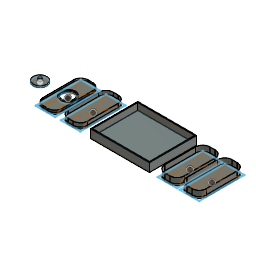
insert_test (Autodesk Fusion 360 design; units mm, degrees)
Autodesk Fusion 360 part; units mm, degrees
sketch "Sketch1" plane through (0, 0, 0) normal (0, 1, 0) x (1, 0, 0)
  line L0 (163.5, 131) -> (-163.5, 131)
  line L1 (-163.5, 131) -> (-163.5, -131)
  line L2 (-163.5, -131) -> (163.5, -131)
  line L3 (163.5, -131) -> (163.5, 131)
  line L4 (163.5, 131) -> (-163.5, -131) construction
  line L5 (-163.5, 131) -> (163.5, -131) construction
  line L6 (158.5, 126) -> (-158.5, 126)
  line L7 (-158.5, 126) -> (-158.5, -126)
  line L8 (-158.5, -126) -> (158.5, -126)
  line L9 (158.5, -126) -> (158.5, 126)
  line L10 (158.5, 126) -> (-158.5, -126) construction
  line L11 (-158.5, 126) -> (158.5, -126) construction
  dimension "d1" = 327
  dimension "d2" = 262
  dimension "d3" = 317
  dimension "d4" = 252
  constraint horizontal L0
  constraint perpendicular L0 L1
  constraint parallel L0 L2
  constraint parallel L1 L3
  constraint coincident L4 origin
  constraint coincident L5 origin
  constraint horizontal L6
  constraint perpendicular L6 L7
  constraint parallel L6 L8
  constraint parallel L7 L9
  constraint coincident L10 origin
  constraint coincident L11 origin
  measures "d1" distance of L1.end L2.end
  measures "d2" distance of L0.end L1.end
  measures "d3" distance of L7.end L8.end
  measures "d4" distance of L6.end L7.end
extrude "Extrude1" add sketch "Sketch1" along normal blind 48 makes body 1
sketch "Sketch2" plane through (0, 0, 0) normal (0, 1, 0) x (1, 0, 0)
  line L0 (-161.5, 130) -> (161.5, 130)
  line L1 (161.5, 130) -> (161.5, -130)
  line L2 (161.5, -130) -> (-161.5, -130)
  line L3 (-161.5, -130) -> (-161.5, 130)
  line L4 (-161.5, 130) -> (161.5, -130) construction
  line L5 (161.5, 130) -> (-161.5, -130) construction
  dimension "d7" = 323
  dimension "d8" = 260
  constraint horizontal L0
  constraint perpendicular L0 L1
  constraint parallel L0 L2
  constraint parallel L1 L3
  constraint coincident L4 origin
  constraint coincident L5 origin
  measures "d7" distance of L1.end L2.end
  measures "d8" distance of L0.end L1.end
extrude "Extrude2" add sketch "Sketch2" along normal blind 10 bodies 1
sketch "Sketch3" plane through (0, 10, 0) normal (0, 1, 0) x (-1, 0, 0)
  line L0 (158.5, 126) -> (-158.5, 126)
  line L1 (-158.5, 126) -> (-158.5, -126)
  line L2 (-158.5, -126) -> (158.5, -126)
  line L3 (158.5, -126) -> (158.5, 126)
sketch "Sketch4" plane through (0, 10, 0) normal (0, 1, 0) x (-1, 0, 0)
  line L0 (158.5, 126) -> (-158.5, 126)
  line L1 (-158.5, 126) -> (-158.5, -126)
  line L2 (-158.5, -126) -> (158.5, -126)
  line L3 (158.5, -126) -> (158.5, 126)
  line L4 (-320, -124) -> (-220, -124)
  line L5 (-220, -124) -> (-220, 124)
  line L6 (-220, 124) -> (-320, 124)
  line L7 (-320, 124) -> (-320, -124)
  line L8 (-320, -124) -> (-220, 124) construction
  line L9 (-220, -124) -> (-320, 124) construction
  point P0 (-270, 0)
  dimension "d17" = 100
  dimension "d18" = 248
  constraint horizontal L4
  constraint perpendicular L4 L5
  constraint parallel L4 L6
  constraint parallel L5 L7
  constraint coincident L8 P0
  constraint coincident L9 P0
  measures "d17" distance of L5.end L6.end
  measures "d18" distance of L4.end L5.end
sketch "Sketch5" plane through (0, 20, 0) normal (0, 1, 0) x (-1, 0, 0)
sketch "Sketch6" plane through (0, 10, 0) normal (0, 1, 0) x (-1, 0, 0)
  line L0 (158.5, 126) -> (-158.5, 126)
  line L1 (-158.5, 126) -> (-158.5, -126)
  line L2 (-158.5, -126) -> (158.5, -126)
  line L3 (158.5, -126) -> (158.5, 126)
sketch "Sketch9" plane through (0, 20, 0) normal (0, 1, 0) x (-1, 0, 0)
sketch "Sketch10" plane through (0, 10, 0) normal (0, 1, 0) x (-1, 0, 0)
sketch "Sketch11" plane through (0, 0, 0) normal (0, 1, 0) x (1, 0, 0)
sketch "Sketch12" plane through (0, 20, 0) normal (0, 1, 0) x (1, 0, 0)
sketch "Sketch14" plane through (0, 0, 0) normal (0, 1, 0) x (1, 0, 0)
sketch "Sketch15" plane through (0, 0, 0) normal (0, 1, 0) x (1, 0, 0)
  line L0 (207.402, 121.291) -> (316.402, 121.291)
  line L1 (316.402, 121.291) -> (316.402, -130.109)
  line L2 (316.402, -130.109) -> (207.402, -130.109)
  line L3 (207.402, -130.109) -> (207.402, 121.291)
  line L4 (207.402, 121.291) -> (316.402, -130.109) construction
  line L5 (316.402, 121.291) -> (207.402, -130.109) construction
  line L6 (315.802, 120.691) -> (208.002, 120.691)
  line L7 (208.002, 120.691) -> (208.002, -129.509)
  line L8 (208.002, -129.509) -> (315.802, -129.509)
  line L9 (315.802, -129.509) -> (315.802, 120.691)
  line L10 (315.802, 120.691) -> (208.002, -129.509) construction
  line L11 (208.002, 120.691) -> (315.802, -129.509) construction
  point P0 (261.902, -4.409)
  point P1 (261.902, -4.409)
  dimension "d42" = 109
  dimension "d43" = 251.4
  dimension "d44" = 107.8
  dimension "d45" = 250.2
  constraint horizontal L0
  constraint perpendicular L0 L1
  constraint parallel L0 L2
  constraint parallel L1 L3
  constraint coincident L4 P1
  constraint coincident L5 P1
  constraint horizontal L6
  constraint perpendicular L6 L7
  constraint parallel L6 L8
  constraint parallel L7 L9
  constraint coincident L10 P1
  constraint coincident L11 P1
  constraint coincident P1 P0
  measures "d42" distance of L1.end L2.end
  measures "d43" distance of L0.end L1.end
  measures "d44" distance of L7.end L8.end
  measures "d45" distance of L6.end L7.end
extrude "Extrude8" add sketch "Sketch15" along normal blind 40 separate body makes body 2
extrude "Extrude9" add sketch "Sketch15" along normal blind 10 contours L6 L7 L8 L9 bodies 2
sketch "Sketch16" plane through (0, 0, 0) normal (0, 1, 0) x (1, 0, 0)
sketch "Sketch17" plane through (0, 0, 0) normal (0, 1, 0) x (1, 0, 0)
  line L0 (329.9494, 121.3227) -> (438.9494, 121.3227)
  line L1 (438.9494, 121.3227) -> (438.9494, -130.0773)
  line L2 (438.9494, -130.0773) -> (329.9494, -130.0773)
  line L3 (329.9494, -130.0773) -> (329.9494, 121.3227)
  line L4 (329.9494, 121.3227) -> (438.9494, -130.0773) construction
  line L5 (438.9494, 121.3227) -> (329.9494, -130.0773) construction
  line L6 (438.3494, 120.7227) -> (330.5494, 120.7227)
  line L7 (330.5494, 120.7227) -> (330.5494, -129.4773)
  line L8 (330.5494, -129.4773) -> (438.3494, -129.4773)
  line L9 (438.3494, -129.4773) -> (438.3494, 120.7227)
  line L10 (438.3494, 120.7227) -> (330.5494, -129.4773) construction
  line L11 (330.5494, 120.7227) -> (438.3494, -129.4773) construction
  point P0 (384.4494, -4.3773)
  point P1 (384.4494, -4.3773)
  dimension "d50" = 109
  dimension "d51" = 251.4
  dimension "d52" = 107.8
  dimension "d53" = 250.2
  constraint horizontal L0
  constraint perpendicular L0 L1
  constraint parallel L0 L2
  constraint parallel L1 L3
  constraint coincident L4 P1
  constraint coincident L5 P1
  constraint horizontal L6
  constraint perpendicular L6 L7
  constraint parallel L6 L8
  constraint parallel L7 L9
  constraint coincident L10 P1
  constraint coincident L11 P1
  constraint coincident P1 P0
  measures "d50" distance of L1.end L2.end
  measures "d51" distance of L0.end L1.end
  measures "d52" distance of L7.end L8.end
  measures "d53" distance of L6.end L7.end
sketch "Sketch18" plane through (0, 0, 0) normal (0, 1, 0) x (1, 0, 0)
  line L0 (434.5, 120.7) -> (325.5, 120.7)
  line L1 (325.5, 120.7) -> (325.5, -120.7)
  line L2 (325.5, -120.7) -> (434.5, -120.7)
  line L3 (434.5, -120.7) -> (434.5, 120.7)
  line L4 (434.5, 120.7) -> (325.5, -120.7) construction
  line L5 (325.5, 120.7) -> (434.5, -120.7) construction
  point P0 (380, 0)
  dimension "d54" = 109
  dimension "d55" = 241.4
  constraint horizontal L0
  constraint perpendicular L0 L1
  constraint parallel L0 L2
  constraint parallel L1 L3
  constraint coincident L4 P0
  constraint coincident L5 P0
  measures "d54" distance of L1.end L2.end
  measures "d55" distance of L0.end L1.end
sketch "Sketch20" plane through (0, 0, 0) normal (0, 1, 0) x (1, 0, 0)
  line L0 (-225.9, 125.7) -> (-334.5, 125.7)
  line L1 (-334.5, 125.7) -> (-334.5, -125.5)
  line L2 (-334.5, -125.5) -> (-225.9, -125.5)
  line L3 (-225.9, -125.5) -> (-225.9, 125.7)
  line L4 (-225.9, 125.7) -> (-334.5, -125.5) construction
  line L5 (-334.5, 125.7) -> (-225.9, -125.5) construction
  point P0 (-280.2, 0.1)
  dimension "d60" = 108.6
  dimension "d61" = 251.2
  constraint horizontal L0
  constraint perpendicular L0 L1
  constraint parallel L0 L2
  constraint parallel L1 L3
  constraint coincident L4 P0
  constraint coincident L5 P0
  measures "d60" distance of L1.end L2.end
  measures "d61" distance of L0.end L1.end
sketch "Sketch35" plane through (0, 0, 0) normal (0, 1, 0) x (1, 0, 0)
  line L0 (-365.7, 125.7) -> (-474.3, 125.7)
  line L1 (-474.3, 125.7) -> (-474.3, -125.7)
  line L2 (-474.3, -125.7) -> (-365.7, -125.7)
  line L3 (-365.7, -125.7) -> (-365.7, 125.7)
  line L4 (-365.7, 125.7) -> (-474.3, -125.7) construction
  line L5 (-474.3, 125.7) -> (-365.7, -125.7) construction
  circle A0 centre (-420, 0) radius 37.5
  point P0 (-420, 0)
  dimension "d73" = 108.6
  dimension "d82" = 75
  dimension "d111" = 251.4
  constraint horizontal L0
  constraint perpendicular L0 L1
  constraint parallel L0 L2
  constraint parallel L1 L3
  constraint coincident L4 P0
  constraint coincident L5 P0
  constraint coincident P0 A0.centre
  measures "d73" distance of L1.end L2.end
  measures "d82" diameter of A0
  measures "d111" distance of L0.end L1.end
sketch "Sketch37" plane through (0, 0, 0) normal (0, 1, 0) x (1, 0, 0)
  line L0 (-366.8902, 125.3136) -> (-473.6902, 125.3136)
  line L1 (-473.6902, 125.3136) -> (-473.6902, -124.8864)
  line L2 (-473.6902, -124.8864) -> (-366.8902, -124.8864)
  line L3 (-366.8902, -124.8864) -> (-366.8902, 125.3136)
  line L4 (-366.8902, 125.3136) -> (-473.6902, -124.8864) construction
  line L5 (-473.6902, 125.3136) -> (-366.8902, -124.8864) construction
  line L6 (-367.5902, 124.6136) -> (-472.9902, 124.6136)
  line L7 (-472.9902, 124.6136) -> (-472.9902, -124.1864)
  line L8 (-472.9902, -124.1864) -> (-367.5902, -124.1864)
  line L9 (-367.5902, -124.1864) -> (-367.5902, 124.6136)
  line L10 (-367.5902, 124.6136) -> (-472.9902, -124.1864) construction
  line L11 (-472.9902, 124.6136) -> (-367.5902, -124.1864) construction
  point P0 (-420.2902, 0.2136)
  point P1 (-420.2902, 0.2136)
  dimension "d76" = 106.8
  dimension "d77" = 250.2
  dimension "d78" = 105.4
  dimension "d79" = 248.8
  constraint horizontal L0
  constraint perpendicular L0 L1
  constraint parallel L0 L2
  constraint parallel L1 L3
  constraint coincident L4 P1
  constraint coincident L5 P1
  constraint horizontal L6
  constraint perpendicular L6 L7
  constraint parallel L6 L8
  constraint parallel L7 L9
  constraint coincident L10 P1
  constraint coincident L11 P1
  constraint coincident P1 P0
  measures "d76" distance of L1.end L2.end
  measures "d77" distance of L0.end L1.end
  measures "d78" distance of L7.end L8.end
  measures "d79" distance of L6.end L7.end
extrude "Extrude14" add sketch "Sketch37" along normal blind 20 separate body makes body 3
sketch "Sketch38" plane through (0, 0, 0) normal (0, 1, 0) x (1, 0, 0)
extrude "Extrude15" add sketch "Sketch35" along normal blind 10 bodies 3
sketch "Sketch39" plane through (0, 0, 0) normal (0, 1, 0) x (1, 0, 0)
sketch "Sketch40" plane through (0, 0, 0) normal (0, 0, 1) x (1, 0, 0)
sketch "Sketch41" plane through (0, 0, 0) normal (0, 1, 0) x (1, 0, 0)
sketch "Sketch42" plane through (0, 0, 0) normal (0, 1, 0) x (1, 0, 0)
  line L0 (-226.5, 125.1) -> (-333.9, 125.1)
  line L1 (-333.9, 125.1) -> (-333.9, -125.1)
  line L2 (-333.9, -125.1) -> (-226.5, -125.1)
  line L3 (-226.5, -125.1) -> (-226.5, 125.1)
  line L4 (-226.5, 125.1) -> (-333.9, -125.1) construction
  line L5 (-333.9, 125.1) -> (-226.5, -125.1) construction
  line L6 (-225.8538, 125.6801) -> (-334.5462, 125.6801)
  line L7 (-334.5462, 125.6801) -> (-334.5462, -125.6801)
  line L8 (-334.5462, -125.6801) -> (-225.8538, -125.6801)
  line L9 (-225.8538, -125.6801) -> (-225.8538, 125.6801)
  line L10 (-225.8538, 125.6801) -> (-334.5462, -125.6801) construction
  line L11 (-334.5462, 125.6801) -> (-225.8538, -125.6801) construction
  point P0 (-280.2, 0)
  point P1 (-280.2, 0)
  dimension "d85" = 107.4
  dimension "d86" = 250.2
  constraint horizontal L0
  constraint perpendicular L0 L1
  constraint parallel L0 L2
  constraint parallel L1 L3
  constraint coincident L4 P1
  constraint coincident L5 P1
  constraint horizontal L6
  constraint perpendicular L6 L7
  constraint parallel L6 L8
  constraint parallel L7 L9
  constraint coincident L10 P1
  constraint coincident L11 P1
  constraint coincident P1 P0
  measures "d85" distance of L1.end L2.end
  measures "d86" distance of L0.end L1.end
sketch "Sketch43" plane through (0, 0, 0) normal (0, 1, 0) x (1, 0, 0)
sketch "Sketch44" plane through (0, 0, 0) normal (0, 1, 0) x (1, 0, 0)
sketch "Sketch45" plane through (0, 10, 0) normal (0, 1, 0) x (-1, 0, 0)
  circle A0 centre (420, 0) radius 37.5
  line L0 (367.5902, -124.6136) -> (472.9902, -124.6136)
  line L1 (472.9902, -124.6136) -> (472.9902, 124.1864)
  line L2 (472.9902, 124.1864) -> (367.5902, 124.1864)
  line L3 (367.5902, 124.1864) -> (367.5902, -124.6136)
  circle A1 centre (420, 0) radius 40
  circle A2 centre (420, 0) radius 35
  dimension "d91" = 80
  dimension "d92" = 70
  constraint concentric A0 A1
  constraint concentric A0 A2
  measures "d91" diameter of A1
  measures "d92" diameter of A2
extrude "Extrude18" add sketch "Sketch45" along normal blind 5 contours A0 | A1 bodies 3
sketch "Sketch46" plane through (0, 0, 0) normal (0, 0, 1) x (1, 0, 0)
sketch "Sketch47" plane through (0, 0, 0) normal (0, 1, 0) x (1, 0, 0)
sketch "Sketch48" plane through (0, 0, 0) normal (0, 1, 0) x (1, 0, 0)
  circle A0 centre (-575, 0) radius 37.2
  circle A1 centre (-575, 0) radius 10
  dimension "d95" = 74.4
  dimension "d96" = 20
  constraint concentric A0 A1
  measures "d95" diameter of A0
  measures "d96" diameter of A1
extrude "Extrude19" add sketch "Sketch48" along normal blind 25 separate body contours A1 makes body 4
sketch "Sketch49" plane through (0, 0, 0) normal (0, 1, 0) x (1, 0, 0)
extrude "Extrude20" add sketch "Sketch48" along normal blind 9.6 bodies 4
fillet "Fillet1" radius 3 1 edges at (-584.3233, 25, 3.6162) on bodies 4
extrude "Extrude23" add sketch "Sketch17" along normal blind 40 separate body makes body 5
extrude "Extrude24" add sketch "Sketch17" along normal blind 10 contours L6 L7 L8 L9 bodies 5
extrude "Extrude25" add sketch "Sketch42" along normal blind 30 separate body makes body 6
extrude "Extrude26" add sketch "Sketch42" along normal blind 10 contours L0 L1 L2 L3 bodies 6
fillet "Fillet2" radius 40 1 edges at (-472.9902, 15, -124.6136) on bodies 3
fillet "Fillet3" radius 40 1 edges at (-367.5902, 15, -124.6136) on bodies 3
fillet "Fillet4" radius 40 1 edges at (-226.5, 20, -125.1) on bodies 6
fillet "Fillet5" radius 40 1 edges at (-333.9, 20, -125.1) on bodies 6
fillet "Fillet6" radius 40 1 edges at (-472.9902, 15, 124.1864) on bodies 3
fillet "Fillet7" radius 40 1 edges at (-367.5902, 15, 124.1864) on bodies 3
fillet "Fillet8" radius 40 1 edges at (-226.5, 20, 125.1) on bodies 6
fillet "Fillet9" radius 40 1 edges at (-333.9, 20, 125.1) on bodies 6
fillet "Fillet10" radius 40 1 edges at (208.002, 25, -120.691) on bodies 2
fillet "Fillet11" radius 40 1 edges at (315.802, 25, -120.691) on bodies 2
fillet "Fillet12" radius 40 1 edges at (438.3494, 25, -120.7227) on bodies 5
fillet "Fillet13" radius 40 1 edges at (330.5494, 25, -120.7227) on bodies 5
fillet "Fillet14" radius 40 1 edges at (-366.8902, 15, -125.3136) on bodies 3
fillet "Fillet15" radius 40 1 edges at (-365.7, 5, -125.7) on bodies 3
fillet "Fillet16" radius 40 1 edges at (-473.6902, 15, -125.3136) on bodies 3
fillet "Fillet17" radius 40 1 edges at (-474.3, 5, -125.7) on bodies 3
fillet "Fillet18" radius 40 1 edges at (-473.6902, 15, 124.8864) on bodies 3
fillet "Fillet19" radius 40 1 edges at (-474.3, 5, 125.7) on bodies 3
fillet "Fillet20" radius 40 1 edges at (-366.8902, 15, 124.8864) on bodies 3
fillet "Fillet21" radius 40 1 edges at (-365.7, 5, 125.7) on bodies 3
fillet "Fillet22" radius 40 1 edges at (-225.8538, 15, 125.6801) on bodies 6
fillet "Fillet23" radius 40 1 edges at (-334.5462, 15, 125.6801) on bodies 6
fillet "Fillet24" radius 40 1 edges at (-334.5462, 15, -125.6801) on bodies 6
fillet "Fillet25" radius 40 1 edges at (-225.8538, 15, -125.6801) on bodies 6
fillet "Fillet26" radius 40 1 edges at (207.402, 20, -121.291) on bodies 2
fillet "Fillet27" radius 40 1 edges at (316.402, 20, -121.291) on bodies 2
fillet "Fillet28" radius 40 1 edges at (329.9494, 20, -121.3227) on bodies 5
fillet "Fillet29" radius 40 1 edges at (438.9494, 20, -121.3227) on bodies 5
fillet "Fillet30" radius 40 1 edges at (208.002, 25, 129.509) on bodies 2
fillet "Fillet31" radius 40 1 edges at (315.802, 25, 129.509) on bodies 2
fillet "Fillet32" radius 40 1 edges at (438.3494, 25, 129.4773) on bodies 5
fillet "Fillet33" radius 40 1 edges at (330.5494, 25, 129.4773) on bodies 5
fillet "Fillet34" radius 40 1 edges at (207.402, 20, 130.109) on bodies 2
fillet "Fillet35" radius 40 1 edges at (329.9494, 20, 130.0773) on bodies 5
fillet "Fillet36" radius 40 1 edges at (316.402, 20, 130.109) on bodies 2
fillet "Fillet37" radius 40 1 edges at (438.9494, 20, 130.0773) on bodies 5
equation "d76 = 108 mm - 1.2 mm"
equation "d78 = 106.8 mm - 1.4 mm"
equation "d79 = 250.2 mm - 1.4 mm"
